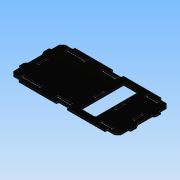
# Autodesk Inventor part: AK-C-C10-Main-Board
Saved by Autodesk Inventor 2016 (Build 200138000, 138)
## iProperties
Created: 2016-03-30
Part Number: AK-C-C10-Main-Board
Material: Generic
Document SubType Name: Modeling
Designer: admin
Density: 1 g/cm^3
Appearance: Anodized - Black
Author: admin
Autodesk Inventor part; units mm, degrees
ref_plane "YZ Plane" through (0, 0, 0) normal (1, 0, 0) x (0, 1, 0)
ref_plane "XZ Plane" through (0, 0, 0) normal (0, 1, 0) x (-1, 0, 0)
ref_plane "XY Plane" through (0, 0, 0) normal (0, 0, 1) x (1, 0, 0)
derived "AK-C-C10-Top.ipt"
sketch "Sketch2_1" plane through (15.9674, 83.4048, 10) normal (0, 0, -1) x (1, 0, 0)
  line L0 (111, 31.525) -> (111, 24.3742)
  line L1 (111, 24.3742) -> (113, 21.6242)
  line L2 (113, 21.6242) -> (113, 15.7)
  line L3 (113, 15.7) -> (111, 15.7)
  line L4 (111, 15.7) -> (111, 13.7)
  line L5 (111, 13.7) -> (113, 13.7)
  line L6 (113, 13.7) -> (113, 11.7)
  line L7 (113, 11.7) -> (111, 11.7)
  line L8 (111, 11.7) -> (111, 9.7)
  line L9 (111, 9.7) -> (113, 9.7)
  line L10 (113, 9.7) -> (113, 7.3)
  line L11 (113, 7.3) -> (110.4678, 7.3)
  arc A0 (110.4678, 7.3) -> (110.1142, 6.4464) centre (110.4678, 6.8) ccw
  line L12 (110.1142, 6.4464) -> (110.6118, 5.9489)
  arc A1 (109.5511, 4.8882) -> (110.6118, 5.9489) centre (111, 4.5) ccw
  line L13 (109.5511, 4.8882) -> (109.0536, 5.3858)
  arc A2 (109.0536, 5.3858) -> (108.2, 5.0322) centre (108.7, 5.0322) ccw
  line L14 (108.2, 5.0322) -> (108.2, 2.3)
  line L15 (108.2, 2.3) -> (106.2, 2.3)
  line L16 (106.2, 2.3) -> (106.2, 4.5)
  line L17 (106.2, 4.5) -> (104.2, 4.5)
  line L18 (104.2, 4.5) -> (104.2, 2.3)
  line L19 (104.2, 2.3) -> (102.2, 2.3)
  line L20 (102.2, 2.3) -> (102.2, 4.5)
  line L21 (102.2, 4.5) -> (100.2, 4.5)
  line L22 (100.2, 4.5) -> (100.2, 2.3)
  line L23 (100.2, 2.3) -> (60.5, 2.3)
  line L24 (60.5, 2.3) -> (60.5, 4.5)
  line L25 (60.5, 4.5) -> (58.5, 4.5)
  line L26 (58.5, 4.5) -> (58.5, 2.3)
  line L27 (58.5, 2.3) -> (56.5, 2.3)
  line L28 (56.5, 2.3) -> (56.5, 4.5)
  line L29 (56.5, 4.5) -> (54.5, 4.5)
  line L30 (54.5, 4.5) -> (54.5, 2.3)
  line L31 (54.5, 2.3) -> (52.5, 2.3)
  line L32 (52.5, 2.3) -> (52.5, 4.5)
  line L33 (52.5, 4.5) -> (50.5, 4.5)
  line L34 (50.5, 4.5) -> (50.5, 2.3)
  line L35 (50.5, 2.3) -> (10.8, 2.3)
  line L36 (10.8, 2.3) -> (10.8, 4.5)
  line L37 (10.8, 4.5) -> (8.8, 4.5)
  line L38 (8.8, 4.5) -> (8.8, 2.3)
  line L39 (8.8, 2.3) -> (6.8, 2.3)
  line L40 (6.8, 2.3) -> (6.8, 4.5)
  line L41 (6.8, 4.5) -> (4.8, 4.5)
  line L42 (4.8, 4.5) -> (4.8, 2.3)
  line L43 (4.8, 2.3) -> (2.8, 2.3)
  line L44 (2.8, 2.3) -> (2.8, 5.0322)
  arc A3 (2.8, 5.0322) -> (1.9464, 5.3858) centre (2.3, 5.0322) ccw
  line L45 (1.9464, 5.3858) -> (1.4489, 4.8882)
  arc A4 (0.3882, 5.9489) -> (1.4489, 4.8882) centre (0, 4.5) ccw
  line L46 (0.3882, 5.9489) -> (0.8858, 6.4464)
  arc A5 (0.8858, 6.4464) -> (0.5322, 7.3) centre (0.5322, 6.8) ccw
  line L47 (0.5322, 7.3) -> (-2, 7.3)
  line L48 (-2, 7.3) -> (-2, 9.7)
  line L49 (-2, 9.7) -> (0, 9.7)
  line L50 (0, 9.7) -> (0, 11.7)
  line L51 (0, 11.7) -> (-2, 11.7)
  line L52 (-2, 11.7) -> (-2, 13.7)
  line L53 (-2, 13.7) -> (0, 13.7)
  line L54 (0, 13.7) -> (0, 15.7)
  line L55 (0, 15.7) -> (-2, 15.7)
  line L56 (-2, 15.7) -> (-2, 23.3362)
  line L57 (-2, 23.3362) -> (0, 26.7706)
  line L58 (0, 26.7706) -> (0, 31.525)
  line L59 (0, 31.525) -> (-1.5, 31.525)
  line L60 (-1.5, 31.525) -> (-1.5, 30.1864)
  arc A6 (-3, 30.1864) -> (-1.5, 30.1864) centre (-2.25, 29.525) ccw
  line L61 (-3, 30.1864) -> (-3, 31.525)
  line L62 (-3, 31.525) -> (-4.5, 31.525)
  line L63 (-4.5, 31.525) -> (-4.5, 4.5)
  arc A7 (-4.5, 4.5) -> (0, 0) centre (0, 4.5) ccw
  line L64 (0, 0) -> (111, 0)
  arc A8 (111, 0) -> (115.5, 4.5) centre (111, 4.5) ccw
  line L65 (115.5, 4.5) -> (115.5, 31.525)
  line L66 (115.5, 31.525) -> (114, 31.525)
  line L67 (114, 31.525) -> (114, 32.8636)
  arc A9 (114, 32.8636) -> (112.5, 32.8636) centre (113.25, 33.525) ccw
  line L68 (112.5, 32.8636) -> (112.5, 31.525)
  line L69 (112.5, 31.525) -> (111, 31.525)
  point P0 (55.5, 31.525)
sketch "Sketch3" plane through (126.9674, 20.3548, 10) normal (0, 0, -1) x (-1, 0, 0)
  line L0 (111, 31.525) -> (111, 24.3742)
  line L1 (111, 24.3742) -> (113, 21.6242)
  line L2 (113, 21.6242) -> (113, 15.7)
  line L3 (113, 15.7) -> (111, 15.7)
  line L4 (111, 15.7) -> (111, 13.7)
  line L5 (111, 13.7) -> (113, 13.7)
  line L6 (113, 13.7) -> (113, 11.7)
  line L7 (113, 11.7) -> (111, 11.7)
  line L8 (111, 11.7) -> (111, 9.7)
  line L9 (111, 9.7) -> (113, 9.7)
  line L10 (113, 9.7) -> (113, 7.3)
  line L11 (113, 7.3) -> (110.4678, 7.3)
  arc A0 (110.4678, 7.3) -> (110.1142, 6.4464) centre (110.4678, 6.8) ccw
  line L12 (110.1142, 6.4464) -> (110.6118, 5.9489)
  arc A1 (109.5511, 4.8882) -> (110.6118, 5.9489) centre (111, 4.5) ccw
  line L13 (109.5511, 4.8882) -> (109.0536, 5.3858)
  arc A2 (109.0536, 5.3858) -> (108.2, 5.0322) centre (108.7, 5.0322) ccw
  line L14 (108.2, 5.0322) -> (108.2, 2.3)
  line L15 (108.2, 2.3) -> (106.2, 2.3)
  line L16 (106.2, 2.3) -> (106.2, 4.5)
  line L17 (106.2, 4.5) -> (104.2, 4.5)
  line L18 (104.2, 4.5) -> (104.2, 2.3)
  line L19 (104.2, 2.3) -> (102.2, 2.3)
  line L20 (102.2, 2.3) -> (102.2, 4.5)
  line L21 (102.2, 4.5) -> (100.2, 4.5)
  line L22 (100.2, 4.5) -> (100.2, 2.3)
  line L23 (100.2, 2.3) -> (60.5, 2.3)
  line L24 (60.5, 2.3) -> (60.5, 4.5)
  line L25 (60.5, 4.5) -> (58.5, 4.5)
  line L26 (58.5, 4.5) -> (58.5, 2.3)
  line L27 (58.5, 2.3) -> (56.5, 2.3)
  line L28 (56.5, 2.3) -> (56.5, 4.5)
  line L29 (56.5, 4.5) -> (54.5, 4.5)
  line L30 (54.5, 4.5) -> (54.5, 2.3)
  line L31 (54.5, 2.3) -> (52.5, 2.3)
  line L32 (52.5, 2.3) -> (52.5, 4.5)
  line L33 (52.5, 4.5) -> (50.5, 4.5)
  line L34 (50.5, 4.5) -> (50.5, 2.3)
  line L35 (50.5, 2.3) -> (10.8, 2.3)
  line L36 (10.8, 2.3) -> (10.8, 4.5)
  line L37 (10.8, 4.5) -> (8.8, 4.5)
  line L38 (8.8, 4.5) -> (8.8, 2.3)
  line L39 (8.8, 2.3) -> (6.8, 2.3)
  line L40 (6.8, 2.3) -> (6.8, 4.5)
  line L41 (6.8, 4.5) -> (4.8, 4.5)
  line L42 (4.8, 4.5) -> (4.8, 2.3)
  line L43 (4.8, 2.3) -> (2.8, 2.3)
  line L44 (2.8, 2.3) -> (2.8, 5.0322)
  arc A3 (2.8, 5.0322) -> (1.9464, 5.3858) centre (2.3, 5.0322) ccw
  line L45 (1.9464, 5.3858) -> (1.4489, 4.8882)
  arc A4 (0.3882, 5.9489) -> (1.4489, 4.8882) centre (0, 4.5) ccw
  line L46 (0.3882, 5.9489) -> (0.8858, 6.4464)
  arc A5 (0.8858, 6.4464) -> (0.5322, 7.3) centre (0.5322, 6.8) ccw
  line L47 (0.5322, 7.3) -> (-2, 7.3)
  line L48 (-2, 7.3) -> (-2, 9.7)
  line L49 (-2, 9.7) -> (0, 9.7)
  line L50 (0, 9.7) -> (0, 11.7)
  line L51 (0, 11.7) -> (-2, 11.7)
  line L52 (-2, 11.7) -> (-2, 13.7)
  line L53 (-2, 13.7) -> (0, 13.7)
  line L54 (0, 13.7) -> (0, 15.7)
  line L55 (0, 15.7) -> (-2, 15.7)
  line L56 (-2, 15.7) -> (-2, 23.3362)
  line L57 (-2, 23.3362) -> (0, 26.7706)
  line L58 (0, 26.7706) -> (0, 31.525)
  line L59 (0, 31.525) -> (-1.5, 31.525)
  line L60 (-1.5, 31.525) -> (-1.5, 30.1864)
  arc A6 (-3, 30.1864) -> (-1.5, 30.1864) centre (-2.25, 29.525) ccw
  line L61 (-3, 30.1864) -> (-3, 31.525)
  line L62 (-3, 31.525) -> (-4.5, 31.525)
  line L63 (-4.5, 31.525) -> (-4.5, 4.5)
  arc A7 (-4.5, 4.5) -> (0, 0) centre (0, 4.5) ccw
  line L64 (0, 0) -> (111, 0)
  arc A8 (111, 0) -> (115.5, 4.5) centre (111, 4.5) ccw
  line L65 (115.5, 4.5) -> (115.5, 31.525)
  line L66 (115.5, 31.525) -> (114, 31.525)
  line L67 (114, 31.525) -> (114, 32.8636)
  arc A9 (114, 32.8636) -> (112.5, 32.8636) centre (113.25, 33.525) ccw
  line L68 (112.5, 32.8636) -> (112.5, 31.525)
  line L69 (112.5, 31.525) -> (111, 31.525)
  point P0 (55.5, 31.525)
sketch "Sketch5" plane through (126.9674, 83.4048, 0) normal (0, 0, -1) x (-1, 0, 0)
  line L0 (29, -9.525) -> (42, -9.525)
  line L1 (43, -10.525) -> (43, -52.525)
  line L2 (42, -53.525) -> (29, -53.525)
  line L3 (28, -52.525) -> (28, -10.525)
  arc A0 (29, -9.525) -> (28, -10.525) centre (29, -10.525) ccw
  arc A1 (43, -10.525) -> (42, -9.525) centre (42, -10.525) ccw
  arc A2 (28, -52.525) -> (29, -53.525) centre (29, -52.525) ccw
  arc A3 (42, -53.525) -> (43, -52.525) centre (42, -52.525) ccw
  line L4 (64.4102, -31.525) -> (104.2401, -31.525) construction
  line L5 (85.2044, -44.525) -> (93.2044, -44.525)
  line L6 (93.2044, -44.525) -> (93.2044, -52.525)
  line L7 (93.2044, -52.525) -> (85.2044, -52.525)
  line L8 (85.2044, -52.525) -> (85.2044, -44.525)
  line L9 (85.2044, -27.525) -> (93.2044, -27.525)
  line L10 (93.2044, -27.525) -> (93.2044, -35.525)
  line L11 (93.2044, -35.525) -> (85.2044, -35.525)
  line L12 (85.2044, -35.525) -> (85.2044, -27.525)
  line L13 (85.2044, -10.525) -> (93.2044, -10.525)
  line L14 (93.2044, -10.525) -> (93.2044, -18.525)
  line L15 (93.2044, -18.525) -> (85.2044, -18.525)
  line L16 (85.2044, -18.525) -> (85.2044, -10.525)
  line L17 (99.2044, -44.525) -> (107.2044, -44.525)
  line L18 (107.2044, -44.525) -> (107.2044, -52.525)
  line L19 (107.2044, -52.525) -> (99.2044, -52.525)
  line L20 (99.2044, -52.525) -> (99.2044, -44.525)
  line L21 (99.2044, -27.525) -> (107.2044, -27.525)
  line L22 (107.2044, -27.525) -> (107.2044, -35.525)
  line L23 (107.2044, -35.525) -> (99.2044, -35.525)
  line L24 (99.2044, -35.525) -> (99.2044, -27.525)
  line L25 (99.2044, -10.525) -> (107.2044, -10.525)
  line L26 (107.2044, -10.525) -> (107.2044, -18.525)
  line L27 (107.2044, -18.525) -> (99.2044, -18.525)
  line L28 (99.2044, -18.525) -> (99.2044, -10.525)
  line L29 (45.5684, -14.525) -> (74.4446, -14.525) construction
  line L30 (56.1088, -11.525) -> (80.1088, -11.525)
  line L31 (80.6088, -12.025) -> (80.6088, -51.025)
  line L32 (80.1088, -51.525) -> (56.1088, -51.525)
  line L33 (55.6088, -51.025) -> (55.6088, -12.025)
  arc A4 (56.1088, -11.525) -> (55.6088, -12.025) centre (56.1088, -12.025) ccw
  arc A5 (80.6088, -12.025) -> (80.1088, -11.525) centre (80.1088, -12.025) ccw
  arc A6 (55.6088, -51.025) -> (56.1088, -51.525) centre (56.1088, -51.025) ccw
  arc A7 (80.1088, -51.525) -> (80.6088, -51.025) centre (80.1088, -51.025) ccw
  circle A8 centre (111, -58.55) radius 3
  circle A9 centre (0, -4.5) radius 3
  circle A10 centre (0, -58.55) radius 3
  circle A11 centre (111, -4.5) radius 3
  line L34 (111, 0) -> (0, 0)
  arc A12 (0, 0) -> (-4.5, -4.5) centre (0, -4.5) ccw
  line L35 (-4.5, -4.5) -> (-4.5, -58.55)
  arc A13 (-4.5, -58.55) -> (0, -63.05) centre (0, -58.55) ccw
  line L36 (0, -63.05) -> (111, -63.05)
  arc A14 (111, -63.05) -> (115.5, -58.55) centre (111, -58.55) ccw
  line L37 (115.5, -58.55) -> (115.5, -4.5)
  arc A15 (115.5, -4.5) -> (111, 0) centre (111, -4.5) ccw
  line L38 (-2, -51.35) -> (-2, -49.35)
  line L39 (-2, -9.7) -> (-2, -7.3)
  point P0 (54.886, -31.525)
  point P1 (85.2044, -14.525)
  point P2 (115.5, -31.525)
sketch "Sketch6" plane through (0, 0, 0) normal (0, 0, 1) x (1, 0, 0)
  line L0 (123.221, 78.4048) -> (116.6674, 78.4048)
  line L1 (115.6674, 79.4048) -> (115.6674, 80.6048)
  line L2 (115.6674, 80.6048) -> (76.9674, 80.6048)
  line L3 (76.9674, 80.6048) -> (76.9674, 79.4048)
  line L4 (75.9674, 78.4048) -> (66.9674, 78.4048)
  line L5 (65.9674, 79.4048) -> (65.9674, 80.6048)
  line L6 (65.9674, 80.6048) -> (27.2674, 80.6048)
  line L7 (27.2674, 80.6048) -> (27.2674, 79.4048)
  line L8 (26.2674, 78.4048) -> (19.7139, 78.4048)
  line L9 (16.4674, 75.1584) -> (16.4674, 68.2048)
  line L10 (15.4674, 67.2048) -> (14.4674, 67.2048)
  line L11 (14.4674, 67.2048) -> (14.4674, 61.1972)
  line L12 (14.4674, 61.1972) -> (16.3316, 57.9961)
  line L13 (16.4674, 57.4928) -> (16.4674, 44.0416)
  line L14 (16.2762, 43.4534) -> (14.4674, 40.9664)
  line L15 (14.4674, 40.9664) -> (14.4674, 36.5548)
  line L16 (14.4674, 36.5548) -> (15.4674, 36.5548)
  line L17 (16.4674, 35.5548) -> (16.4674, 28.6013)
  line L18 (19.7139, 25.3548) -> (26.2674, 25.3548)
  line L19 (27.2674, 24.3548) -> (27.2674, 23.1548)
  line L20 (27.2674, 23.1548) -> (65.9674, 23.1548)
  line L21 (65.9674, 23.1548) -> (65.9674, 24.3548)
  line L22 (66.9674, 25.3548) -> (75.9674, 25.3548)
  line L23 (76.9674, 24.3548) -> (76.9674, 23.1548)
  line L24 (115.6674, 23.1548) -> (115.6674, 24.3548)
  line L25 (116.6674, 25.3548) -> (123.221, 25.3548)
  line L26 (126.4674, 28.6013) -> (126.4674, 35.5548)
  line L27 (127.4674, 36.5548) -> (128.4674, 36.5548)
  line L28 (128.4674, 36.5548) -> (128.4674, 42.5625)
  line L29 (128.4674, 42.5625) -> (126.6033, 45.7636)
  line L30 (126.4674, 46.2668) -> (126.4674, 59.7181)
  line L31 (126.6587, 60.3063) -> (128.4674, 62.7933)
  line L32 (128.4674, 62.7933) -> (128.4674, 67.2048)
  line L33 (128.4674, 67.2048) -> (127.4674, 67.2048)
  line L34 (126.4674, 68.2048) -> (126.4674, 75.1584)
  line L35 (116.1674, 81.1048) -> (76.4674, 81.1048) projected
  line L36 (116.1674, 78.9048) -> (116.1674, 81.1048) projected
  line L37 (118.1674, 78.9048) -> (116.1674, 78.9048) projected
  line L38 (118.1674, 81.1048) -> (118.1674, 78.9048) projected
  line L39 (120.1674, 81.1048) -> (118.1674, 81.1048) projected
  line L40 (120.1674, 78.9048) -> (120.1674, 81.1048) projected
  line L41 (122.1674, 78.9048) -> (120.1674, 78.9048) projected
  line L42 (122.1674, 81.1048) -> (122.1674, 78.9048) projected
  line L43 (124.1674, 81.1048) -> (122.1674, 81.1048) projected
  line L44 (124.1674, 78.3726) -> (124.1674, 81.1048) projected
  arc A0 (124.1674, 78.3726) -> (125.021, 78.019) centre (124.6674, 78.3726) ccw projected
  arc A1 (126.0817, 76.9584) -> (126.4352, 76.1048) centre (126.4352, 76.6048) ccw projected
  line L45 (128.9674, 76.1048) -> (126.4352, 76.1048) projected
  line L46 (128.9674, 73.7048) -> (128.9674, 76.1048) projected
  line L47 (126.9674, 71.7048) -> (126.9674, 73.7048) projected
  line L48 (128.9674, 71.7048) -> (126.9674, 71.7048) projected
  line L49 (126.9674, 73.7048) -> (128.9674, 73.7048) projected
  line L50 (126.9674, 67.7048) -> (126.9674, 69.7048) projected
  line L51 (128.9674, 67.7048) -> (126.9674, 67.7048) projected
  line L52 (128.9674, 61.7806) -> (128.9674, 67.7048) projected
  line L53 (126.9674, 59.0306) -> (128.9674, 61.7806) projected
  line L54 (126.9674, 51.8798) -> (126.9674, 59.0306) projected
  line L55 (126.9674, 47.1254) -> (126.9674, 51.8798) projected
  line L56 (128.9674, 43.6911) -> (126.9674, 47.1254) projected
  line L57 (128.9674, 36.0548) -> (128.9674, 43.6911) projected
  line L58 (126.9674, 36.0548) -> (128.9674, 36.0548) projected
  line L59 (126.9674, 34.0548) -> (126.9674, 36.0548) projected
  line L60 (128.9674, 34.0548) -> (126.9674, 34.0548) projected
  line L61 (128.9674, 32.0548) -> (128.9674, 34.0548) projected
  line L62 (126.9674, 32.0548) -> (128.9674, 32.0548) projected
  line L63 (126.9674, 30.0548) -> (126.9674, 32.0548) projected
  line L64 (128.9674, 30.0548) -> (126.9674, 30.0548) projected
  line L65 (128.9674, 27.6548) -> (128.9674, 30.0548) projected
  line L66 (126.4352, 27.6548) -> (128.9674, 27.6548) projected
  arc A2 (126.4352, 27.6548) -> (126.0817, 26.8013) centre (126.4352, 27.1548) ccw projected
  arc A3 (125.021, 25.7406) -> (124.1674, 25.3871) centre (124.6674, 25.3871) ccw projected
  line L67 (124.1674, 22.6548) -> (124.1674, 25.3871) projected
  line L68 (122.1674, 22.6548) -> (124.1674, 22.6548) projected
  line L69 (122.1674, 24.8548) -> (122.1674, 22.6548) projected
  line L70 (120.1674, 24.8548) -> (122.1674, 24.8548) projected
  line L71 (120.1674, 22.6548) -> (120.1674, 24.8548) projected
  line L72 (118.1674, 22.6548) -> (120.1674, 22.6548) projected
  line L73 (118.1674, 24.8548) -> (118.1674, 22.6548) projected
  line L74 (116.1674, 24.8548) -> (118.1674, 24.8548) projected
  line L75 (116.1674, 22.6548) -> (116.1674, 24.8548) projected
  line L76 (76.4674, 22.6548) -> (116.1674, 22.6548) projected
  line L77 (76.4674, 24.8548) -> (76.4674, 22.6548) projected
  line L78 (74.4674, 24.8548) -> (76.4674, 24.8548) projected
  line L79 (74.4674, 22.6548) -> (74.4674, 24.8548) projected
  line L80 (72.4674, 22.6548) -> (74.4674, 22.6548) projected
  line L81 (72.4674, 24.8548) -> (72.4674, 22.6548) projected
  line L82 (70.4674, 24.8548) -> (72.4674, 24.8548) projected
  line L83 (70.4674, 22.6548) -> (70.4674, 24.8548) projected
  line L84 (68.4674, 22.6548) -> (70.4674, 22.6548) projected
  line L85 (68.4674, 24.8548) -> (68.4674, 22.6548) projected
  line L86 (66.4674, 24.8548) -> (68.4674, 24.8548) projected
  line L87 (66.4674, 22.6548) -> (66.4674, 24.8548) projected
  line L88 (26.7674, 22.6548) -> (66.4674, 22.6548) projected
  line L89 (26.7674, 24.8548) -> (26.7674, 22.6548) projected
  line L90 (24.7674, 24.8548) -> (26.7674, 24.8548) projected
  line L91 (24.7674, 22.6548) -> (24.7674, 24.8548) projected
  line L92 (22.7674, 22.6548) -> (24.7674, 22.6548) projected
  line L93 (22.7674, 24.8548) -> (22.7674, 22.6548) projected
  line L94 (20.7674, 24.8548) -> (22.7674, 24.8548) projected
  line L95 (20.7674, 22.6548) -> (20.7674, 24.8548) projected
  line L96 (18.7674, 22.6548) -> (20.7674, 22.6548) projected
  line L97 (18.7674, 25.3871) -> (18.7674, 22.6548) projected
  arc A4 (18.7674, 25.3871) -> (17.9139, 25.7406) centre (18.2674, 25.3871) ccw projected
  arc A5 (16.8532, 26.8013) -> (16.4997, 27.6548) centre (16.4997, 27.1548) ccw projected
  line L98 (13.9674, 27.6548) -> (16.4997, 27.6548) projected
  line L99 (13.9674, 30.0548) -> (13.9674, 27.6548) projected
  line L100 (15.9674, 30.0548) -> (13.9674, 30.0548) projected
  line L101 (15.9674, 32.0548) -> (15.9674, 30.0548) projected
  line L102 (13.9674, 32.0548) -> (15.9674, 32.0548) projected
  line L103 (13.9674, 34.0548) -> (13.9674, 32.0548) projected
  line L104 (15.9674, 34.0548) -> (13.9674, 34.0548) projected
  line L105 (15.9674, 36.0548) -> (15.9674, 34.0548) projected
  line L106 (13.9674, 36.0548) -> (15.9674, 36.0548) projected
  line L107 (13.9674, 41.9791) -> (13.9674, 36.0548) projected
  line L108 (15.9674, 44.7291) -> (13.9674, 41.9791) projected
  line L109 (15.9674, 51.8798) -> (15.9674, 44.7291) projected
  line L110 (15.9674, 56.6342) -> (15.9674, 51.8798) projected
  line L111 (13.9674, 60.0686) -> (15.9674, 56.6342) projected
  line L112 (13.9674, 67.7048) -> (13.9674, 60.0686) projected
  line L113 (15.9674, 67.7048) -> (13.9674, 67.7048) projected
  line L114 (15.9674, 69.7048) -> (15.9674, 67.7048) projected
  line L115 (13.9674, 69.7048) -> (15.9674, 69.7048) projected
  line L116 (13.9674, 71.7048) -> (13.9674, 69.7048) projected
  line L117 (15.9674, 71.7048) -> (13.9674, 71.7048) projected
  line L118 (15.9674, 73.7048) -> (15.9674, 71.7048) projected
  line L119 (13.9674, 73.7048) -> (15.9674, 73.7048) projected
  line L120 (13.9674, 76.1048) -> (13.9674, 73.7048) projected
  line L121 (16.4997, 76.1048) -> (13.9674, 76.1048) projected
  arc A6 (16.4997, 76.1048) -> (16.8532, 76.9584) centre (16.4997, 76.6048) ccw projected
  arc A7 (17.9139, 78.019) -> (18.7674, 78.3726) centre (18.2674, 78.3726) ccw projected
  line L122 (18.7674, 81.1048) -> (18.7674, 78.3726) projected
  line L123 (20.7674, 81.1048) -> (18.7674, 81.1048) projected
  line L124 (20.7674, 78.9048) -> (20.7674, 81.1048) projected
  line L125 (22.7674, 78.9048) -> (20.7674, 78.9048) projected
  line L126 (22.7674, 81.1048) -> (22.7674, 78.9048) projected
  line L127 (24.7674, 81.1048) -> (22.7674, 81.1048) projected
  line L128 (24.7674, 78.9048) -> (24.7674, 81.1048) projected
  line L129 (26.7674, 78.9048) -> (24.7674, 78.9048) projected
  line L130 (26.7674, 81.1048) -> (26.7674, 78.9048) projected
  line L131 (66.4674, 81.1048) -> (26.7674, 81.1048) projected
  line L132 (66.4674, 78.9048) -> (66.4674, 81.1048) projected
  line L133 (68.4674, 78.9048) -> (66.4674, 78.9048) projected
  line L134 (68.4674, 81.1048) -> (68.4674, 78.9048) projected
  line L135 (70.4674, 81.1048) -> (68.4674, 81.1048) projected
  line L136 (70.4674, 78.9048) -> (70.4674, 81.1048) projected
  line L137 (72.4674, 78.9048) -> (70.4674, 78.9048) projected
  line L138 (72.4674, 81.1048) -> (72.4674, 78.9048) projected
  line L139 (74.4674, 81.1048) -> (72.4674, 81.1048) projected
  line L140 (74.4674, 78.9048) -> (74.4674, 81.1048) projected
  line L141 (76.4674, 78.9048) -> (74.4674, 78.9048) projected
  line L142 (76.4674, 81.1048) -> (76.4674, 78.9048) projected
  line L143 (115.6674, 23.1548) -> (76.9674, 23.1548)
  arc A8 (115.6674, 79.4048) -> (116.6674, 78.4048) centre (116.6674, 79.4048) ccw
  arc A9 (75.9674, 78.4048) -> (76.9674, 79.4048) centre (75.9674, 79.4048) ccw
  arc A10 (65.9674, 79.4048) -> (66.9674, 78.4048) centre (66.9674, 79.4048) ccw
  arc A11 (26.2674, 78.4048) -> (27.2674, 79.4048) centre (26.2674, 79.4048) ccw
  arc A12 (15.4674, 67.2048) -> (16.4674, 68.2048) centre (15.4674, 68.2048) ccw
  arc A13 (16.4674, 57.4928) -> (16.3316, 57.9961) centre (15.4674, 57.4928) ccw
  arc A14 (16.2762, 43.4534) -> (16.4674, 44.0416) centre (15.4674, 44.0416) ccw
  arc A15 (16.4674, 35.5548) -> (15.4674, 36.5548) centre (15.4674, 35.5548) ccw
  arc A16 (126.4674, 68.2048) -> (127.4674, 67.2048) centre (127.4674, 68.2048) ccw
  arc A17 (126.6587, 60.3063) -> (126.4674, 59.7181) centre (127.4674, 59.7181) ccw
  arc A18 (126.4674, 46.2668) -> (126.6033, 45.7636) centre (127.4674, 46.2668) ccw
  arc A19 (127.4674, 36.5548) -> (126.4674, 35.5548) centre (127.4674, 35.5548) ccw
  arc A20 (116.6674, 25.3548) -> (115.6674, 24.3548) centre (116.6674, 24.3548) ccw
  arc A21 (76.9674, 24.3548) -> (75.9674, 25.3548) centre (75.9674, 24.3548) ccw
  arc A22 (66.9674, 25.3548) -> (65.9674, 24.3548) centre (66.9674, 24.3548) ccw
  arc A23 (27.2674, 24.3548) -> (26.2674, 25.3548) centre (26.2674, 24.3548) ccw
  line L144 (126.4674, 75.1584) -> (123.221, 78.4048)
  line L145 (126.4674, 28.6013) -> (123.221, 25.3548)
  line L146 (19.7139, 25.3548) -> (16.4674, 28.6013)
  line L147 (19.7139, 78.4048) -> (16.4674, 75.1584)
  point P0 (0, 0)
  point P1 (76.9674, 78.4048)
  point P2 (65.9674, 78.4048)
  point P3 (27.2674, 25.3548)
  point P4 (65.9674, 25.3548)
  point P5 (76.9674, 25.3548)
  point P6 (126.4674, 67.2048)
  dimension "d1" = 0.5
  dimension "d2" = 0.5
  dimension "d3" = 0.5
  dimension "d4" = 0.5
  dimension "d5" = 0.5
  dimension "d7" = 0.5
  dimension "d8" = 0.5
  dimension "d9" = 0.5
  dimension "d10" = 1
  dimension "d11" = 0.5
  dimension "d13" = 1
  dimension "d17" = 0.5
  dimension "d18" = 0.5
  dimension "d19" = 0.5
  dimension "d20" = 0.5
  dimension "d21" = 0.5
  dimension "d22" = 0.5
  dimension "d23" = 1
  dimension "d24" = 1
  dimension "d25" = 1
  dimension "d27" = 0.5
  dimension "d28" = 0.5
  dimension "d33" = 0.5
  dimension "d34" = 45
  constraints: 80 end point, 32 point on circle, 32 tangent, 27 point on line, 16 centre point, 16 perpendicular, 15 equal radius, 9 parallel, 7 collinear, 3 horizontal, 2 horizontal alignment, 1 vertical, 1 vertical alignment
  measures "d1" distance between parallel lines of L2 L35
  measures "d2" distance between parallel lines of L142 L3
  measures "d3" distance between parallel lines of L4 L141
  measures "d4" distance between parallel lines of L132 L5
  measures "d5" distance between parallel lines of L130 L7
  measures "d7" distance between parallel lines of L118 L9
  measures "d8" distance between parallel lines of L113 L10
  measures "d9" distance between parallel lines of L112 L11
  measures "d10" distance between parallel lines of L111 L12
  measures "d11" distance between parallel lines of L109 L13
  measures "d13" distance between parallel lines of L108 L14
  measures "d17" distance between parallel lines of L94 L18
  measures "d18" distance between parallel lines of L88 L20
  measures "d19" distance between parallel lines of L24 L75
  measures "d20" distance between parallel lines of L26 L63
  measures "d21" distance between parallel lines of L28 L57
  measures "d22" distance between parallel lines of L30 L54
  measures "d23" distance between parallel lines of L29 L56
  measures "d24" distance between parallel lines of L31 L53
  measures "d25" radius of A8
  measures "d27" distance between parallel lines of L107 L15
  measures "d28" distance between parallel lines of L106 L16
  measures "d33" distance edge to line of A0 L144
  measures "d34" angle of L34 L144
extrude "Extrusion1" add sketch "Sketch6" against normal blind 1.6
extrude "Extrusion2" cut sketch "Sketch5" along normal up to next contours L0 A1 L1 A3 L2 A2 L3 A0
sketch "Sketch7" plane through (0, 0, 0) normal (0, 0, 1) x (1, 0, 0)
  arc A0 (98.9674, 72.8798) -> (97.9674, 73.8798) centre (97.9674, 72.8798) ccw projected
  line L0 (98.9674, 72.8798) -> (98.9674, 30.8798) projected
  arc A1 (97.9674, 29.8798) -> (98.9674, 30.8798) centre (97.9674, 30.8798) ccw projected
  line L1 (97.9674, 29.8798) -> (84.9674, 29.8798) projected
  arc A2 (83.9674, 30.8798) -> (84.9674, 29.8798) centre (84.9674, 30.8798) ccw projected
  line L2 (83.9674, 30.8798) -> (83.9674, 72.8798) projected
  arc A3 (84.9674, 73.8798) -> (83.9674, 72.8798) centre (84.9674, 72.8798) ccw projected
  line L3 (84.9674, 73.8798) -> (97.9674, 73.8798) projected
  line L4 (123.221, 78.4048) -> (116.6674, 78.4048) projected
  arc A4 (115.6674, 79.4048) -> (116.6674, 78.4048) centre (116.6674, 79.4048) ccw projected
  line L5 (115.6674, 79.4048) -> (115.6674, 80.6048) projected
  line L6 (115.6674, 80.6048) -> (76.9674, 80.6048) projected
  line L7 (76.9674, 80.6048) -> (76.9674, 79.4048) projected
  arc A5 (75.9674, 78.4048) -> (76.9674, 79.4048) centre (75.9674, 79.4048) ccw projected
  line L8 (75.9674, 78.4048) -> (66.9674, 78.4048) projected
  arc A6 (65.9674, 79.4048) -> (66.9674, 78.4048) centre (66.9674, 79.4048) ccw projected
  line L9 (65.9674, 79.4048) -> (65.9674, 80.6048) projected
  line L10 (65.9674, 80.6048) -> (27.2674, 80.6048) projected
  line L11 (27.2674, 80.6048) -> (27.2674, 79.4048) projected
  arc A7 (26.2674, 78.4048) -> (27.2674, 79.4048) centre (26.2674, 79.4048) ccw projected
  line L12 (26.2674, 78.4048) -> (19.7139, 78.4048) projected
  line L13 (19.7139, 78.4048) -> (16.4674, 75.1584) projected
  line L14 (16.4674, 75.1584) -> (16.4674, 68.2048) projected
  arc A8 (15.4674, 67.2048) -> (16.4674, 68.2048) centre (15.4674, 68.2048) ccw projected
  line L15 (15.4674, 67.2048) -> (14.4674, 67.2048) projected
  line L16 (14.4674, 67.2048) -> (14.4674, 61.1972) projected
  line L17 (14.4674, 61.1972) -> (16.3316, 57.9961) projected
  arc A9 (16.4674, 57.4928) -> (16.3316, 57.9961) centre (15.4674, 57.4928) ccw projected
  line L18 (16.4674, 57.4928) -> (16.4674, 44.0416) projected
  arc A10 (16.2762, 43.4534) -> (16.4674, 44.0416) centre (15.4674, 44.0416) ccw projected
  line L19 (16.2762, 43.4534) -> (14.4674, 40.9664) projected
  line L20 (14.4674, 40.9664) -> (14.4674, 36.5548) projected
  line L21 (14.4674, 36.5548) -> (15.4674, 36.5548) projected
  arc A11 (16.4674, 35.5548) -> (15.4674, 36.5548) centre (15.4674, 35.5548) ccw projected
  line L22 (16.4674, 35.5548) -> (16.4674, 28.6013) projected
  line L23 (16.4674, 28.6013) -> (19.7139, 25.3548) projected
  line L24 (19.7139, 25.3548) -> (26.2674, 25.3548) projected
  arc A12 (27.2674, 24.3548) -> (26.2674, 25.3548) centre (26.2674, 24.3548) ccw projected
  line L25 (27.2674, 24.3548) -> (27.2674, 23.1548) projected
  line L26 (27.2674, 23.1548) -> (65.9674, 23.1548) projected
  line L27 (65.9674, 23.1548) -> (65.9674, 24.3548) projected
  arc A13 (66.9674, 25.3548) -> (65.9674, 24.3548) centre (66.9674, 24.3548) ccw projected
  line L28 (66.9674, 25.3548) -> (75.9674, 25.3548) projected
  arc A14 (76.9674, 24.3548) -> (75.9674, 25.3548) centre (75.9674, 24.3548) ccw projected
  line L29 (76.9674, 24.3548) -> (76.9674, 23.1548) projected
  line L30 (76.9674, 23.1548) -> (115.6674, 23.1548) projected
  line L31 (115.6674, 23.1548) -> (115.6674, 24.3548) projected
  arc A15 (116.6674, 25.3548) -> (115.6674, 24.3548) centre (116.6674, 24.3548) ccw projected
  line L32 (116.6674, 25.3548) -> (123.221, 25.3548) projected
  line L33 (123.221, 25.3548) -> (126.4674, 28.6013) projected
  line L34 (126.4674, 28.6013) -> (126.4674, 35.5548) projected
  arc A16 (127.4674, 36.5548) -> (126.4674, 35.5548) centre (127.4674, 35.5548) ccw projected
  line L35 (127.4674, 36.5548) -> (128.4674, 36.5548) projected
  line L36 (128.4674, 36.5548) -> (128.4674, 42.5625) projected
  line L37 (128.4674, 42.5625) -> (126.6033, 45.7636) projected
  arc A17 (126.4674, 46.2668) -> (126.6033, 45.7636) centre (127.4674, 46.2668) ccw projected
  line L38 (126.4674, 46.2668) -> (126.4674, 59.7181) projected
  arc A18 (126.6587, 60.3063) -> (126.4674, 59.7181) centre (127.4674, 59.7181) ccw projected
  line L39 (126.6587, 60.3063) -> (128.4674, 62.7933) projected
  line L40 (128.4674, 62.7933) -> (128.4674, 67.2048) projected
  line L41 (128.4674, 67.2048) -> (127.4674, 67.2048) projected
  arc A19 (126.4674, 68.2048) -> (127.4674, 67.2048) centre (127.4674, 68.2048) ccw projected
  line L42 (126.4674, 68.2048) -> (126.4674, 75.1584) projected
  line L43 (126.4674, 75.1584) -> (123.221, 78.4048) projected
  line L44 (106.4674, 75.9048) -> (117.4674, 75.9048)
  line L45 (118.4674, 75.9048) -> (118.4674, 73.9048)
  line L46 (117.4674, 73.9048) -> (106.4674, 73.9048)
  line L47 (105.4674, 73.9048) -> (105.4674, 75.9048)
  line L48 (74.4674, 73.9048) -> (61.4674, 73.9048)
  line L49 (60.4674, 73.9048) -> (60.4674, 75.9048)
  line L50 (61.4674, 75.9048) -> (74.4674, 75.9048)
  line L51 (75.4674, 75.9048) -> (75.4674, 73.9048)
  line L52 (43.4674, 73.9048) -> (25.4674, 73.9048)
  line L53 (24.4674, 73.9048) -> (24.4674, 75.9048)
  line L54 (25.4674, 75.9048) -> (43.4674, 75.9048)
  line L55 (44.4674, 75.9048) -> (44.4674, 73.9048)
  line L56 (117.4674, 27.8548) -> (106.4674, 27.8548)
  line L57 (105.4674, 27.8548) -> (105.4674, 29.8548)
  line L58 (106.4674, 29.8548) -> (117.4674, 29.8548)
  line L59 (118.4674, 29.8548) -> (118.4674, 27.8548)
  line L60 (74.4674, 27.8548) -> (61.4674, 27.8548)
  line L61 (60.4674, 27.8548) -> (60.4674, 29.8548)
  line L62 (61.4674, 29.8548) -> (74.4674, 29.8548)
  line L63 (75.4674, 29.8548) -> (75.4674, 27.8548)
  line L64 (43.4674, 27.8548) -> (25.4674, 27.8548)
  line L65 (24.4674, 27.8548) -> (24.4674, 29.8548)
  line L66 (25.4674, 29.8548) -> (43.4674, 29.8548)
  line L67 (44.4674, 29.8548) -> (44.4674, 27.8548)
  arc A20 (117.4674, 27.8548) -> (118.4674, 27.8548) centre (117.9674, 27.8548) ccw
  arc A21 (105.4674, 27.8548) -> (106.4674, 27.8548) centre (105.9674, 27.8548) ccw
  arc A22 (118.4674, 29.8548) -> (117.4674, 29.8548) centre (117.9674, 29.8548) ccw
  arc A23 (106.4674, 29.8548) -> (105.4674, 29.8548) centre (105.9674, 29.8548) ccw
  arc A24 (74.4674, 27.8548) -> (75.4674, 27.8548) centre (74.9674, 27.8548) ccw
  arc A25 (75.4674, 29.8548) -> (74.4674, 29.8548) centre (74.9674, 29.8548) ccw
  arc A26 (60.4674, 27.8548) -> (61.4674, 27.8548) centre (60.9674, 27.8548) ccw
  arc A27 (61.4674, 29.8548) -> (60.4674, 29.8548) centre (60.9674, 29.8548) ccw
  arc A28 (43.4674, 27.8548) -> (44.4674, 27.8548) centre (43.9674, 27.8548) ccw
  arc A29 (44.4674, 29.8548) -> (43.4674, 29.8548) centre (43.9674, 29.8548) ccw
  arc A30 (24.4674, 27.8548) -> (25.4674, 27.8548) centre (24.9674, 27.8548) ccw
  arc A31 (25.4674, 29.8548) -> (24.4674, 29.8548) centre (24.9674, 29.8548) ccw
  arc A32 (24.4674, 73.9048) -> (25.4674, 73.9048) centre (24.9674, 73.9048) ccw
  arc A33 (25.4674, 75.9048) -> (24.4674, 75.9048) centre (24.9674, 75.9048) ccw
  arc A34 (44.4674, 75.9048) -> (43.4674, 75.9048) centre (43.9674, 75.9048) ccw
  arc A35 (43.4674, 73.9048) -> (44.4674, 73.9048) centre (43.9674, 73.9048) ccw
  arc A36 (61.4674, 75.9048) -> (60.4674, 75.9048) centre (60.9674, 75.9048) ccw
  arc A37 (60.4674, 73.9048) -> (61.4674, 73.9048) centre (60.9674, 73.9048) ccw
  arc A38 (74.4674, 73.9048) -> (75.4674, 73.9048) centre (74.9674, 73.9048) ccw
  arc A39 (75.4674, 75.9048) -> (74.4674, 75.9048) centre (74.9674, 75.9048) ccw
  arc A40 (105.4674, 73.9048) -> (106.4674, 73.9048) centre (105.9674, 73.9048) ccw
  arc A41 (117.4674, 73.9048) -> (118.4674, 73.9048) centre (117.9674, 73.9048) ccw
  arc A42 (118.4674, 75.9048) -> (117.4674, 75.9048) centre (117.9674, 75.9048) ccw
  arc A43 (106.4674, 75.9048) -> (105.4674, 75.9048) centre (105.9674, 75.9048) ccw
  line L68 (121.7174, 46.8798) -> (120.0174, 46.8798)
  line L69 (120.0174, 47.8798) -> (120.0174, 55.8798)
  line L70 (120.0174, 56.8798) -> (121.7174, 56.8798)
  line L71 (121.7174, 55.8798) -> (121.7174, 47.8798)
  line L72 (102.9674, 46.8798) -> (101.2674, 46.8798)
  line L73 (101.2674, 47.8798) -> (101.2674, 55.8798)
  line L74 (101.2674, 56.8798) -> (102.9674, 56.8798)
  line L75 (102.9674, 55.8798) -> (102.9674, 47.8798)
  line L76 (81.7674, 46.8798) -> (80.0674, 46.8798)
  line L77 (80.0674, 47.8798) -> (80.0674, 55.8798)
  line L78 (80.0674, 56.8798) -> (81.7674, 56.8798)
  line L79 (81.7674, 55.8798) -> (81.7674, 47.8798)
  line L80 (23.6174, 46.8798) -> (21.9174, 46.8798)
  line L81 (21.9174, 47.8798) -> (21.9174, 55.8798)
  line L82 (21.9174, 56.8798) -> (23.6174, 56.8798)
  line L83 (23.6174, 55.8798) -> (23.6174, 47.8798)
  line L84 (78.7082, 51.8798) -> (40.6205, 51.8798) construction
  arc A44 (121.7174, 46.8798) -> (121.7174, 47.8798) centre (121.7174, 47.3798) ccw
  arc A45 (121.7174, 55.8798) -> (121.7174, 56.8798) centre (121.7174, 56.3798) ccw
  arc A46 (120.0174, 56.8798) -> (120.0174, 55.8798) centre (120.0174, 56.3798) ccw
  arc A47 (120.0174, 47.8798) -> (120.0174, 46.8798) centre (120.0174, 47.3798) ccw
  arc A48 (102.9674, 46.8798) -> (102.9674, 47.8798) centre (102.9674, 47.3798) ccw
  arc A49 (102.9674, 55.8798) -> (102.9674, 56.8798) centre (102.9674, 56.3798) ccw
  arc A50 (101.2674, 47.8798) -> (101.2674, 46.8798) centre (101.2674, 47.3798) ccw
  arc A51 (101.2674, 56.8798) -> (101.2674, 55.8798) centre (101.2674, 56.3798) ccw
  arc A52 (81.7674, 46.8798) -> (81.7674, 47.8798) centre (81.7674, 47.3798) ccw
  arc A53 (80.0674, 47.8798) -> (80.0674, 46.8798) centre (80.0674, 47.3798) ccw
  arc A54 (81.7674, 55.8798) -> (81.7674, 56.8798) centre (81.7674, 56.3798) ccw
  arc A55 (80.0674, 56.8798) -> (80.0674, 55.8798) centre (80.0674, 56.3798) ccw
  arc A56 (21.9174, 47.8798) -> (21.9174, 46.8798) centre (21.9174, 47.3798) ccw
  arc A57 (23.6174, 46.8798) -> (23.6174, 47.8798) centre (23.6174, 47.3798) ccw
  arc A58 (23.6174, 55.8798) -> (23.6174, 56.8798) centre (23.6174, 56.3798) ccw
  arc A59 (21.9174, 56.8798) -> (21.9174, 55.8798) centre (21.9174, 56.3798) ccw
  point P0 (0, 0)
  dimension "d39" = 4.7
  dimension "d40" = 2
  dimension "d41" = 13
  dimension "d42" = 8
  dimension "d43" = 30
  dimension "d44" = 15
  dimension "d45" = 16
  dimension "d46" = 20
  dimension "d49" = 4.7
  dimension "d50" = 1
  dimension "d51" = 10
  dimension "d52" = 1.7
  dimension "d53" = 2.3
  dimension "d54" = 17.05
  dimension "d55" = 19.5
  dimension "d56" = 56.45
  constraints: 82 end point, 80 point on circle, 45 point on line, 40 centre point, 40 tangent, 39 equal radius, 18 parallel, 17 collinear, 12 perpendicular, 11 horizontal, 4 other
  measures "d39" distance between parallel lines of L44 L6
  measures "d40" distance of L47.start L47.end
  measures "d41" distance between parallel lines of L45 L47
  measures "d42" distance between parallel lines of L45 L42
  measures "d43" distance between parallel lines of L51 L47
  measures "d44" distance between parallel lines of L49 L51
  measures "d45" distance between parallel lines of L55 L49
  measures "d46" distance of L55.end L53.start
  measures "d49" distance between parallel lines of L56 L30
  measures "d50" diameter of A42
  measures "d51" distance of L70.end L68.start
  measures "d52" distance of L68.start L68.end
  measures "d53" distance between parallel lines of L0 L73
  measures "d54" distance between parallel lines of L75 L69
  measures "d55" distance between parallel lines of L79 L73
  measures "d56" distance between parallel lines of L83 L77
extrude "Extrusion3" cut sketch "Sketch7" against normal blind 1.6 contours L44 A42 L45 A41 L46 A40 L47 A43 | L48 A37 L49 A36 L50 A39 L51 A38 | L52 A32 L53 A33 L54 A34 L55 A35 | L56 A21 L57 A23 L58 A22 L59 A20 | L60 A26 L61 A27 L62 A25 L63 A24 | L64 A30 L65 A31 L66 A29 L67 A28 | L68 A47 L69 A46 L70 A45 L71 A44 | L72 A50 L73 A51 L74 A49 L75 A48 | L76 A53 L77 A55 L78 A54 L79 A52 | L80 A56 L81 A59 L82 A58 L83 A57
equation "\"d2\" = d1"
equation "\"d3\" = d1"
equation "\"d4\" = d1"
equation "\"d5\" = d1"
equation "\"d7\" = d1"
equation "\"d8\" = d7"
equation "\"d9\" = d8"
equation "\"d17\" = d28"
equation "\"d18\" = d17"
equation "\"d19\" = d1"
equation "\"d20\" = d19"
equation "\"d21\" = d1"
equation "\"d22\" = d11"
equation "\"d23\" = d13"
equation "\"d24\" = d23"
equation "\"d27\" = d11"
equation "\"d28\" = d11"
body "Solid1"
